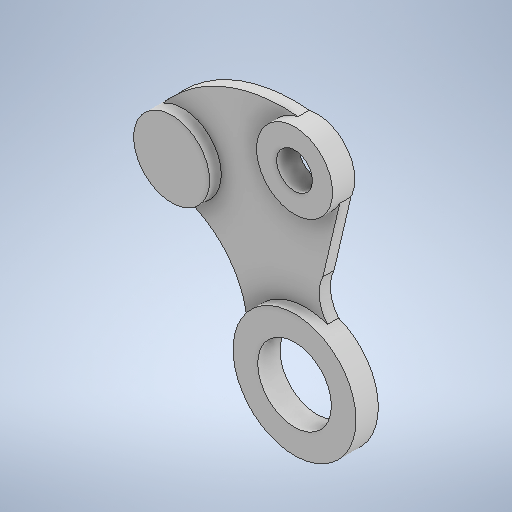
# Autodesk Inventor part: Desafio 2 - MASA - Inventor
Saved by Autodesk Inventor 2025.1 (Build 291241000, 241)
## iProperties
Created: 2025-05-16
Part Number: Desafio 2 - MASA - Inventor
Material: Generic
Document SubType Name: Modeling
Designer: Aluno
Density: 1 g/cm^3
Appearance: Default
Author: Aluno
Autodesk Inventor part; units mm, degrees
ref_plane "YZ Plane" through (0, 0, 0) normal (1, 0, 0) x (0, 1, 0)
ref_plane "XZ Plane" through (0, 0, 0) normal (0, 1, 0) x (-1, 0, 0)
ref_plane "XY Plane" through (0, 0, 0) normal (0, 0, 1) x (1, 0, 0)
sketch "Sketch1" plane through (0, 0, 0) normal (0, 0, 1) x (1, 0, 0)
  circle A0 centre (0, 0) radius 27.5
  circle A1 centre (0, 0) radius 16.5
  circle A2 centre (-55, 60) radius 17
  circle A3 centre (0, 83) radius 17
  circle A4 centre (0, 83) radius 8
  dimension "d0" = 55
  dimension "d1" = 33
  dimension "d2" = 34
  dimension "d3" = 34
  dimension "d4" = 16
  constraints: 5 centre point, 5 coincident
  measures "d0" diameter of A0
  measures "d1" diameter of A1
  measures "d2" diameter of A2
  measures "d3" diameter of A3
  measures "d4" diameter of A4
sketch "Sketch2" plane through (0, 0, 0) normal (0, 0, 1) x (1, 0, 0)
  arc A0 (-3.3945, 99.6876) -> (-63.7995, 74.7841) centre (-10, 30) ccw
  arc A1 (-53.1844, 42.8914) -> (-63.7995, 74.7841) centre (-55, 60) ccw
  arc A2 (-3.3945, 99.6876) -> (15.2517, 75.4247) centre (0, 83) ccw
  arc A3 (10.2232, 25.1691) -> (-26.084, 7.5911) centre (0, 0) ccw
  arc A4 (-26.084, 7.5911) -> (-53.1844, 42.8914) centre (-66, 5) ccw
  arc A5 (7.6702, 43.1174) -> (10.2232, 25.1691) centre (22, 36) ccw
  line L0 (7.6702, 43.1174) -> (15.2517, 75.4247)
  dimension "d8" = 140
  dimension "d9" = 80
  dimension "d10" = 32
  constraints: 12 point on circle, 6 centre point, 2 end point, 1 coincident
  measures "d8" diameter of A0
  measures "d9" diameter of A4
  measures "d10" diameter of A5
extrude "Extrusion1" add sketch "Sketch1" along normal blind 10
extrude "Extrusion2" add sketch "Sketch2" along normal blind 5
body "Solid1"
